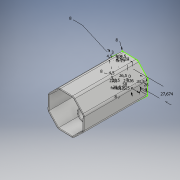
# Autodesk Inventor part: BaseR02
Saved by Autodesk Inventor 2018.1 (Build 221171000, 171)
## iProperties
Created: 2017-10-18
Part Number: BaseR02
Material: Generic
Document SubType Name: Modeling
Designer: s167968
Density: 1 g/cm^3
Appearance: Default
Author: s167968
Autodesk Inventor part; units mm, degrees
ref_plane "YZ Plane" through (0, 0, 0) normal (1, 0, 0) x (0, 1, 0)
ref_plane "XZ Plane" through (0, 0, 0) normal (0, 1, 0) x (-1, 0, 0)
ref_plane "XY Plane" through (0, 0, 0) normal (0, 0, 1) x (1, 0, 0)
sketch "Inner" plane through (0, 0, 0) normal (0, 0, 1) x (1, 0, 0)
  line L0 (-16.42323, -33.408376) -> (-38.125208, -10.562627)
  line L1 (-38.125208, -10.562627) -> (-37.31644, 20.937373)
  line L2 (-37.31644, 20.937373) -> (-14.470691, 42.639351)
  line L3 (-14.470691, 42.639351) -> (17.029309, 41.830583)
  line L4 (17.029309, 41.830583) -> (38.731287, 18.984834)
  line L5 (38.731287, 18.984834) -> (37.922519, -12.515166)
  line L6 (37.922519, -12.515166) -> (15.07677, -34.217145)
  line L7 (15.07677, -34.217145) -> (-16.42323, -33.408376)
  line L8 (38.524291, -16.044544) -> (18.717638, -34.930407)
  line L9 (13.00664, -37.138309) -> (-14.3531, -36.487212)
  line L10 (-19.952608, -34.010148) -> (-38.838471, -14.203496)
  line L11 (-41.046372, -8.492497) -> (-40.395276, 18.867243)
  line L12 (-37.918212, 24.466751) -> (-18.11156, 43.352614)
  line L13 (-12.400561, 45.560515) -> (14.959179, 44.909419)
  line L14 (20.558687, 42.432355) -> (39.44455, 22.625702)
  line L15 (41.652451, 16.914704) -> (41.001355, -10.445037)
  circle A0 centre (0.303039, -20.58346) radius 11.75
  circle A1 centre (0.303039, -20.58346) radius 13.25
  arc A2 (-37.918212, 24.466751) -> (-40.395276, 18.867243) centre (-32.397541, 18.676916) ccw
  arc A3 (-41.046372, -8.492497) -> (-38.838471, -14.203496) centre (-33.048637, -8.682824) ccw
  arc A4 (41.652451, 16.914704) -> (39.44455, 22.625702) centre (33.654715, 17.105031) ccw
  arc A5 (38.524291, -16.044544) -> (41.001355, -10.445037) centre (33.003619, -10.25471) ccw
  arc A6 (-19.952608, -34.010148) -> (-14.3531, -36.487212) centre (-14.162774, -28.489477) ccw
  arc A7 (13.00664, -37.138309) -> (18.717638, -34.930407) centre (13.196967, -29.140573) ccw
  arc A8 (-12.400561, 45.560515) -> (-18.11156, 43.352614) centre (-12.590888, 37.562779) ccw
  arc A9 (20.558687, 42.432355) -> (14.959179, 44.909419) centre (14.768852, 36.911683) ccw
  point P0 (0.303039, 4.211103)
  point P1 (0.303039, 4.211103)
  point P2 (40.922519, -13.757807)
  point P3 (16.31941, -37.217145)
  point P4 (-17.665871, -36.408376)
  point P5 (-41.125208, -11.805268)
  point P6 (-40.31644, 22.180013)
  point P7 (-15.713332, 45.639351)
  point P8 (18.27195, 44.830583)
  point P9 (41.731287, 20.227474)
  dimension "d30" = 31.5
  dimension "d31" = 3
  dimension "d32" = 3
  dimension "d33" = 23.5
  dimension "d38" = 26.5
  dimension "d41" = 8
  dimension "d42" = 8
  dimension "d43" = 8
  dimension "d44" = 8
  dimension "d45" = 13.25
  dimension "d75" = 0
  constraints: 32 end point, 16 point on circle, 16 point on line, 16 tangent, 10 centre point, 4 equal radius, 2 coincident, 34 other
  measures "d30" vertical distance of L4.end L5.end
  measures "d31" horizontal distance of L0.end point (-41.125, -11.805)
  measures "d32" horizontal distance of L1.end point (-40.316, 22.18)
  measures "d33" diameter of A0
  measures "d38" diameter of A1
  measures "d41" radius of A2
  measures "d42" radius of A3
  measures "d43" radius of A6
  measures "d44" radius of A8
  measures "d45" distance from line of L7 A1.centre
  measures "d75" horizontal distance of point (0.303, 4.211) A0.centre
extrude "Extrusion2" [suppressed]
extrude "Extrusion3" [suppressed]
sketch "Inner outline for Extrusion4" plane through (0, 0, 0) normal (0, 0, 1) x (1, 0, 0)
  arc A0 (-37.918212, 24.466751) -> (-40.395276, 18.867243) centre (-32.397541, 18.676916) ccw
  line L0 (-18.11156, 43.352614) -> (-37.918212, 24.466751)
  line L1 (-40.395276, 18.867243) -> (-41.046372, -8.492497)
  arc A1 (-12.400561, 45.560515) -> (-18.11156, 43.352614) centre (-12.590888, 37.562779) ccw
  arc A2 (-41.046372, -8.492497) -> (-38.838471, -14.203496) centre (-33.048637, -8.682824) ccw
  line L2 (14.959179, 44.909419) -> (-12.400561, 45.560515)
  line L3 (-38.838471, -14.203496) -> (-19.952608, -34.010148)
  arc A3 (20.558687, 42.432355) -> (14.959179, 44.909419) centre (14.768852, 36.911683) ccw
  arc A4 (-19.952608, -34.010148) -> (-14.3531, -36.487212) centre (-14.162774, -28.489477) ccw
  line L4 (39.44455, 22.625702) -> (20.558687, 42.432355)
  line L5 (-14.3531, -36.487212) -> (13.00664, -37.138309)
  arc A5 (41.652451, 16.914704) -> (39.44455, 22.625702) centre (33.654715, 17.105031) ccw
  arc A6 (13.00664, -37.138309) -> (18.717638, -34.930407) centre (13.196967, -29.140573) ccw
  line L6 (41.001355, -10.445037) -> (41.652451, 16.914704)
  line L7 (18.717638, -34.930407) -> (38.524291, -16.044544)
  arc A7 (38.524291, -16.044544) -> (41.001355, -10.445037) centre (33.003619, -10.25471) ccw
  line L8 (15.07677, -34.217145) -> (-16.42323, -33.408376)
  line L9 (37.922519, -12.515166) -> (15.07677, -34.217145)
  line L10 (38.731287, 18.984834) -> (37.922519, -12.515166)
  line L11 (17.029309, 41.830583) -> (38.731287, 18.984834)
  line L12 (-14.470691, 42.639351) -> (17.029309, 41.830583)
  line L13 (-37.31644, 20.937373) -> (-14.470691, 42.639351)
  line L14 (-38.125208, -10.562627) -> (-37.31644, 20.937373)
  line L15 (-16.42323, -33.408376) -> (-38.125208, -10.562627)
extrude "Extrusion4" add sketch "Inner outline for Extrusion4" along normal blind 145
extrude "Extrusion5" [suppressed]
sketch "Inner outline for Extrusion6" plane through (0, 0, 0) normal (0, 0, 1) x (1, 0, 0)
  line L0 (-16.42323, -33.408376) -> (-38.125208, -10.562627)
  line L1 (15.07677, -34.217145) -> (-16.42323, -33.408376)
  line L2 (-38.125208, -10.562627) -> (-37.31644, 20.937373)
  line L3 (37.922519, -12.515166) -> (15.07677, -34.217145)
  line L4 (-37.31644, 20.937373) -> (-14.470691, 42.639351)
  line L5 (38.731287, 18.984834) -> (37.922519, -12.515166)
  line L6 (-14.470691, 42.639351) -> (17.029309, 41.830583)
  line L7 (17.029309, 41.830583) -> (38.731287, 18.984834)
  circle A0 centre (0.303039, -20.58346) radius 11.75
extrude "Extrusion6" add sketch "Inner outline for Extrusion6" along normal blind 5
sketch "Sketch4" plane through (0, 0, 5) normal (0, 0, 1) x (1, 0, 0)
  line L0 (-29, 27.674) -> (29, 27.674)
  line L1 (29, 27.674) -> (29, 23.174)
  line L2 (29, 23.174) -> (-29, 23.174)
  line L3 (-29, 23.174) -> (-29, 27.674)
  line L4 (-29, -2.826) -> (29, -2.826)
  line L5 (29, -2.826) -> (29, -7.326)
  line L6 (29, -7.326) -> (-29, -7.326)
  line L7 (-29, -7.326) -> (-29, -2.826)
  line L8 (-12, 27.674) -> (12, 27.674)
  line L9 (12, 27.674) -> (12, 32.174)
  line L10 (12, 32.174) -> (-12, 32.174)
  line L11 (-12, 32.174) -> (-12, 27.674)
  line L12 (-12, 36.674) -> (12, 36.674)
  line L13 (12, 36.674) -> (12, 41.174)
  line L14 (12, 41.174) -> (-12, 41.174)
  line L15 (-12, 41.174) -> (-12, 36.674)
  line L16 (-38.125208, -10.562627) -> (-37.31644, 20.937373)
  line L17 (-38.125208, -10.562627) -> (-37.31644, 20.937373)
  circle A0 centre (0, -20.575679) radius 11.75
  circle A1 centre (0, -20.575679) radius 13.25
  line L18 (15.07677, -34.217145) -> (-16.42323, -33.408376)
  point P0 (0, 0)
  dimension "d46" = 58
  dimension "d47" = 4.5
  dimension "d48" = 4.5
  dimension "d49" = 26
  dimension "d52" = 4.5
  dimension "d53" = 24
  dimension "d54" = 12
  dimension "d55" = 4.5
  dimension "d56" = 4.5
  dimension "d57" = 29
  dimension "d58" = 27.674
  dimension "d61" = 23.5
  dimension "d62" = 26.5
  dimension "d73" = 13.25
  dimension "d74" = 2.826
  dimension "d76" = 0
  constraints: 34 end point, 9 equal length, 4 horizontal, 4 perpendicular, 4 point on line, 2 centre point, 1 coincident
  measures "d46" distance of L5.end L6.end
  measures "d47" distance of L2.end L0.start
  measures "d48" distance of L6.end L4.start
  measures "d49" distance between parallel lines of L4 L2
  measures "d52" distance between parallel lines of L12 L10
  measures "d53" distance of L9.end L10.end
  measures "d54" distance from line of L11 point (0, 0)
  measures "d55" distance of L10.end L8.start
  measures "d56" distance of L14.end L12.start
  measures "d57" distance from line of L3 point (0, 0)
  measures "d58" distance from line of point (0, 0) L8
  measures "d61" diameter of A0
  measures "d62" diameter of A1
  measures "d73" distance from line of L18 A0.centre
  measures "d74" distance from line of point (0, 0) L4
  measures "d76" horizontal distance of A0.centre point (0, 0)
extrude "Extrusion7" add sketch "Sketch4" along normal blind 40 contours L0 L1 L2 L3 | L4 L5 L6 L7
extrude "Extrusion8" add sketch "Sketch4" along normal blind 30 contours L11 L10 L9 L0 | L15 L14 L13 L12
sketch "Sketch4 outline for Extrusion9" plane through (0, 0, 5) normal (0, 0, 1) x (1, 0, 0)
  circle A0 centre (0, -20.575679) radius 13.25
  circle A1 centre (0, -20.575679) radius 11.75
extrude "Extrusion9" add sketch "Sketch4 outline for Extrusion9" along normal blind 100
fillet "Fillet1" radius 1 1 edges at (-11.75, -20.5757, 105)
fillet "Fillet2" radius 1 24 edges at (38.3269, 3.2348, 145) (27.8803, 30.4077, 145) (1.2793, 42.235, 145) (-25.8936, 31.7884, 145) (-37.7208, 5.1874, 145) (-0.6732, -33.8128, 145) (26.4996, -23.3662, 145) (-27.2742, -21.9855, 145) (-17.3992, -35.8056, 145) (-0.6732, -36.8128, 145) (16.0817, -36.6024, 145) (28.621, -25.4875, 145) (40.3197, -13.4911, 145) (41.3269, 3.2348, 145) (41.1165, 19.9898, 145) (30.0016, 32.529, 145) (18.0053, 44.2278, 145) (1.2793, 45.235, 145) (-15.4756, 45.0246, 145) (-28.0149, 33.9097, 145) (-39.7136, 21.9134, 145) (-40.7208, 5.1874, 145) (-40.5104, -11.5676, 145) (-29.3955, -24.1068, 145)
equation "\"d45\" = 0.5 * d38"
equation "\"d54\" = 0.5 * d53"
equation "\"d56\" = d55"
equation "\"d57\" = 0.5 * d46"
equation "\"d73\" = d45"
body "Solid2"
